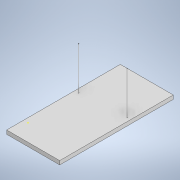
# Autodesk Inventor part: mousetrap
Saved by Autodesk Inventor 2021 (Build 250183000, 183)
## iProperties
Created: 2021-02-20
Part Number: mousetrap
Material: Generic
Document SubType Name: Modeling
Designer: bagal
Density: 1 g/cm^3
Appearance: Default
Author: bagal
Autodesk Inventor part; units mm, degrees
ref_plane "YZ Plane" through (0, 0, 0) normal (1, 0, 0) x (0, 1, 0)
ref_plane "XZ Plane" through (0, 0, 0) normal (0, 1, 0) x (-1, 0, 0)
ref_plane "XY Plane" through (0, 0, 0) normal (0, 0, 1) x (1, 0, 0)
sketch "Sketch1" plane through (0, 0, 0) normal (0, 1, 0) x (-1, 0, 0)
  line L0 (3.9475, 13.9735) -> (3.9475, -81.2765)
  line L1 (3.9475, -81.2765) -> (-40.5025, -81.2765)
  line L2 (-40.5025, -81.2765) -> (-40.5025, 13.9735)
  line L3 (-40.5025, 13.9735) -> (3.9475, 13.9735)
  point P0 (0, 0)
  dimension "d0" = 95.25
  dimension "d1" = 44.45
  dimension "d2" = 95.25
  constraints: 8 end point, 2 perpendicular, 1 vertical
  measures "d0" distance of L0.start L0.end
  measures "d1" distance of L0.end L1.end
  measures "d2" distance of L1.end L2.end
extrude "Extrusion1" add sketch "Sketch1" along normal blind 3.175
sketch "Sketch2" plane through (0, 3.175, 0) normal (0, 1, 0) x (1, 0, 0)
  point P0 (0, 0)
sketch "Sketch3" plane through (0, 3.175, 0) normal (0, 1, 0) x (1, 0, 0)
  line L0 (-3.9475, 81.2765) -> (-3.9475, -13.9735) projected
  line L1 (-3.9475, 81.2765) -> (-0.7725, 81.2765)
  line L2 (40.5025, 81.2765) -> (-3.9475, 81.2765) projected
  line L3 (-0.7725, 81.2765) -> (-0.7725, 43.1765)
  circle A0 centre (-0.7725, 43.1765) radius 0.254
  point P0 (0, 0)
  dimension "d5" = 3.175
  dimension "d6" = 38.1
  dimension "d7" = 0.508
  constraints: 4 end point, 1 centre point, 1 coincident, 1 perpendicular, 1 point on line
  measures "d5" distance of L0.start L1.end
  measures "d6" distance of L1.end L3.end
  measures "d7" diameter of A0
extrude "Extrusion2" add sketch "Sketch3" along normal blind 35.56
sketch "Sketch4" plane through (0, 3.175, 0) normal (0, 1, 0) x (1, 0, 0)
  line L0 (40.5025, 81.2765) -> (-3.9475, 81.2765) projected
  line L1 (40.5025, 81.2765) -> (37.3275, 81.2765)
  line L2 (37.3275, 81.2765) -> (37.3275, 45.7165)
  circle A0 centre (37.3275, 45.7165) radius 0.254
  point P0 (0, 0)
  dimension "d10" = 3.175
  dimension "d11" = 35.56
  dimension "d12" = 0.508
  constraints: 4 end point, 1 centre point, 1 coincident, 1 perpendicular, 1 point on line
  measures "d10" distance of L0.start L1.end
  measures "d11" distance of L1.end L2.end
  measures "d12" diameter of A0
extrude "Extrusion3" add sketch "Sketch4" along normal blind 35.56
sketch "Sketch5" plane through (-0.7725, 38.735, -43.1765) normal (0, 1, 0) x (1, 0, 0)
  line L0 (0, 0) -> (-0.254, 0)
  line L1 (-0.127, 0) -> (-0.127, 0.1164)
  line L2 (-0.127, 0.1164) -> (0.1178, 0.1164)
  line L3 (0.1178, 0.1164) -> (0.1178, -0.1303)
  line L4 (0.1178, -0.1303) -> (-0.127, -0.1303)
  line L5 (-0.127, -0.1303) -> (-0.127, 0)
  point P0 (0.7725, -43.1765)
  dimension "d15" = 0.254
  constraints: 12 end point, 4 perpendicular, 1 horizontal, 1 midpoint, 1 point on line, 1 vertical
  measures "d15" distance of L0.start L0.end
extrude "Extrusion4" add sketch "Sketch5" along normal blind 0.254
body "Solid1"
